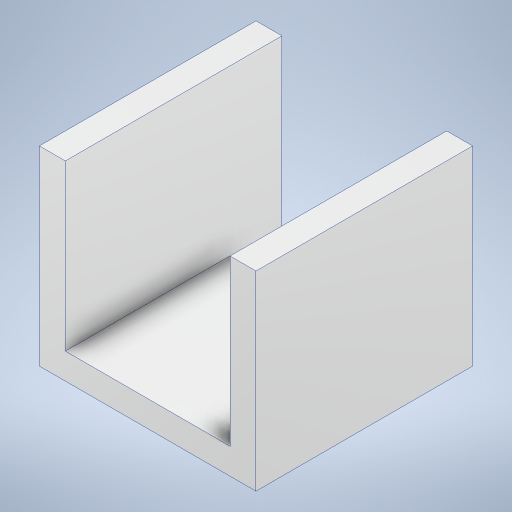
# Autodesk Inventor part: BEARING AND MAGNET DISC MOUNT BRACKET
Saved by Autodesk Inventor 2023 (Build 270158000, 158)
## iProperties
Created: 2022-09-14
Part Number: BEARING AND MAGNET DISC MOUNT BRACKET
Material: Aluminum 6061
Document SubType Name: Modeling
Designer: D.C. Eksteen
Density: 2.7 g/cm^3
Appearance: Aluminum - Flat
Author: D.C. Eksteen
Autodesk Inventor part; units mm, degrees
ref_plane "YZ Plane" through (0, 0, 0) normal (1, 0, 0) x (0, 1, 0)
ref_plane "XZ Plane" through (0, 0, 0) normal (0, 1, 0) x (-1, 0, 0)
ref_plane "XY Plane" through (0, 0, 0) normal (0, 0, 1) x (1, 0, 0)
sketch "Sketch1" plane through (0, 0, 0) normal (0, 0, 1) x (1, 0, 0)
  line L0 (0, 0) -> (-25, 0)
  line L1 (-25, 0) -> (-25, 25)
  line L2 (-25, 25) -> (0, 25)
  line L3 (0, 25) -> (0, 0)
  line L4 (-3, 22) -> (-22, 22)
  line L5 (-22, 22) -> (-22, 3)
  line L6 (-22, 3) -> (-3, 3)
  line L7 (-3, 3) -> (-3, 22)
  line L8 (-22, 22) -> (-25, 22)
  line L9 (-3, 22) -> (0, 22)
  dimension "d0" = 25
  dimension "d1" = 25
  dimension "d2" = 3
  constraints: 20 end point, 4 parallel, 3 perpendicular, 3 point on line, 1 horizontal, 3 other
  measures "d0" distance of L1.end L2.end
  measures "d1" distance of L0.end L1.end
  measures "d2" distance between parallel lines of L2 L4
extrude "Extrusion1" add sketch "Sketch1" along normal blind 25 contours L0 L1 L8 L5 L6 L7 L9 L3
body "Solid1"
